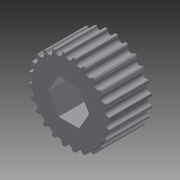
# Autodesk Inventor part: 24t Tooth Pulley .375 Hex Bore 3mm GT2
Saved by Autodesk Inventor 2013 (Build 170138000, 138)
## iProperties
Created: 2013-04-02
Part Number: 24t Tooth Pulley .375 Hex Bore 3mm GT2
Material: Generic
Document SubType Name: Modeling
Designer: mvarma
Density: 1 g/cm^3
Author: mvarma
Autodesk Inventor part; units mm, degrees
ref_plane "YZ Plane" through (0, 0, 0) normal (1, 0, 0) x (0, 1, 0)
ref_plane "XZ Plane" through (0, 0, 0) normal (0, 1, 0) x (-1, 0, 0)
sketch "Sketch1" plane through (0, 0, 0) normal (0, 0, 1) x (1, 0, 0)
  arc A0 (4.5197, -1.1407) -> (6.1695, -2.0932) centre (5.437, -1.4568) ccw
  arc A1 (4.5197, -1.1407) -> (4.3966, -0.6901) centre (4.2781, -0.9646) ccw
  arc A2 (4.3966, -0.6901) -> (4.0923, -0.564) centre (0, -10.8741) ccw
  arc A3 (4.0923, -0.564) -> (3.6866, -0.7956) centre (3.982, -0.8419) ccw
  arc A4 (1.8465, -0.3026) -> (3.6866, -0.7956) centre (2.8144, -0.3705) ccw
  arc A5 (1.8465, -0.3026) -> (1.611, 0.1008) centre (1.5675, -0.195) ccw
  arc A6 (1.611, 0.1008) -> (1.2844, 0.1438) centre (0, -10.8741) ccw
  arc A7 (1.2844, 0.1438) -> (0.9525, -0.1849) centre (1.2498, -0.1532) ccw
  arc A8 (-0.9525, -0.1849) -> (0.9525, -0.1849) centre (0, 0) ccw
  arc A9 (-0.9525, -0.1849) -> (-1.2844, 0.1438) centre (-1.2498, -0.1532) ccw
  arc A10 (-1.2844, 0.1438) -> (-1.611, 0.1008) centre (0, -10.8741) ccw
  arc A11 (-1.611, 0.1008) -> (-1.8465, -0.3026) centre (-1.5675, -0.195) ccw
  arc A12 (-3.6866, -0.7956) -> (-1.8465, -0.3026) centre (-2.8144, -0.3705) ccw
  arc A13 (-3.6866, -0.7956) -> (-4.0923, -0.564) centre (-3.982, -0.8419) ccw
  arc A14 (-4.0923, -0.564) -> (-4.3966, -0.6901) centre (0, -10.8741) ccw
  arc A15 (-4.3966, -0.6901) -> (-4.5197, -1.1407) centre (-4.2781, -0.9646) ccw
  arc A16 (-6.1695, -2.0932) -> (-4.5197, -1.1407) centre (-5.437, -1.4568) ccw
  arc A17 (-6.1695, -2.0932) -> (-6.6213, -1.9745) centre (-6.4428, -2.2144) ccw
  arc A18 (-6.6213, -1.9745) -> (-6.8826, -2.175) centre (0, -10.8741) ccw
  arc A19 (-6.8826, -2.175) -> (-6.8849, -2.6422) centre (-6.6971, -2.4095) ccw
  arc A20 (-8.2319, -3.9892) -> (-6.8849, -2.6422) centre (-7.6891, -3.1849) ccw
  arc A21 (-8.2319, -3.9892) -> (-8.6991, -3.9915) centre (-8.4646, -4.177) ccw
  arc A22 (-8.6991, -3.9915) -> (-8.8996, -4.2528) centre (0, -10.8741) ccw
  arc A23 (-8.8996, -4.2528) -> (-8.7808, -4.7046) centre (-8.6597, -4.4312) ccw
  arc A24 (-9.7333, -6.3544) -> (-8.7808, -4.7046) centre (-9.4172, -5.437) ccw
  arc A25 (-9.7333, -6.3544) -> (-10.184, -6.4775) centre (-9.9095, -6.596) ccw
  arc A26 (-10.184, -6.4775) -> (-10.31, -6.7818) centre (0, -10.8741) ccw
  arc A27 (-10.31, -6.7818) -> (-10.0784, -7.1875) centre (-10.0321, -6.8921) ccw
  arc A28 (-10.5715, -9.0275) -> (-10.0784, -7.1875) centre (-10.5035, -8.0596) ccw
  arc A29 (-10.5715, -9.0275) -> (-10.9749, -9.2631) centre (-10.6791, -9.3065) ccw
  arc A30 (-10.9749, -9.2631) -> (-11.0179, -9.5896) centre (0, -10.8741) ccw
  arc A31 (-11.0179, -9.5896) -> (-10.6892, -9.9216) centre (-10.7209, -9.6242) ccw
  arc A32 (-10.6892, -11.8266) -> (-10.6892, -9.9216) centre (-10.8741, -10.8741) ccw
  arc A33 (-10.6892, -11.8266) -> (-11.0179, -12.1585) centre (-10.7209, -12.1239) ccw
  arc A34 (-11.0179, -12.1585) -> (-10.9749, -12.485) centre (0, -10.8741) ccw
  arc A35 (-10.9749, -12.485) -> (-10.5715, -12.7206) centre (-10.6791, -12.4416) ccw
  arc A36 (-10.0784, -14.5607) -> (-10.5715, -12.7206) centre (-10.5035, -13.6885) ccw
  arc A37 (-10.0784, -14.5607) -> (-10.31, -14.9664) centre (-10.0321, -14.8561) ccw
  arc A38 (-10.31, -14.9664) -> (-10.184, -15.2707) centre (0, -10.8741) ccw
  arc A39 (-10.184, -15.2707) -> (-9.7333, -15.3938) centre (-9.9095, -15.1521) ccw
  arc A40 (-8.7808, -17.0435) -> (-9.7333, -15.3938) centre (-9.4172, -16.3111) ccw
  arc A41 (-8.7808, -17.0435) -> (-8.8996, -17.4954) centre (-8.6597, -17.3169) ccw
  arc A42 (-8.8996, -17.4954) -> (-8.6991, -17.7566) centre (0, -10.8741) ccw
  arc A43 (-8.6991, -17.7566) -> (-8.2319, -17.7589) centre (-8.4646, -17.5711) ccw
  arc A44 (-6.8849, -19.106) -> (-8.2319, -17.7589) centre (-7.6891, -18.5632) ccw
  arc A45 (-6.8849, -19.106) -> (-6.8826, -19.5731) centre (-6.6971, -19.3386) ccw
  arc A46 (-6.8826, -19.5731) -> (-6.6213, -19.7736) centre (0, -10.8741) ccw
  arc A47 (-6.6213, -19.7736) -> (-6.1695, -19.6549) centre (-6.4428, -19.5337) ccw
  arc A48 (-4.5197, -20.6074) -> (-6.1695, -19.6549) centre (-5.437, -20.2913) ccw
  arc A49 (-4.5197, -20.6074) -> (-4.3966, -21.058) centre (-4.2781, -20.7835) ccw
  arc A50 (-4.3966, -21.058) -> (-4.0923, -21.1841) centre (0, -10.8741) ccw
  arc A51 (-4.0923, -21.1841) -> (-3.6866, -20.9525) centre (-3.982, -20.9062) ccw
  arc A52 (-1.8465, -21.4455) -> (-3.6866, -20.9525) centre (-2.8144, -21.3776) ccw
  arc A53 (-1.8465, -21.4455) -> (-1.611, -21.849) centre (-1.5675, -21.5531) ccw
  arc A54 (-1.611, -21.849) -> (-1.2844, -21.8919) centre (0, -10.8741) ccw
  arc A55 (-1.2844, -21.8919) -> (-0.9525, -21.5632) centre (-1.2498, -21.595) ccw
  arc A56 (0.9525, -21.5632) -> (-0.9525, -21.5632) centre (0, -21.7481) ccw
  arc A57 (0.9525, -21.5632) -> (1.2844, -21.8919) centre (1.2498, -21.595) ccw
  arc A58 (1.2844, -21.8919) -> (1.611, -21.849) centre (0, -10.8741) ccw
  arc A59 (1.611, -21.849) -> (1.8465, -21.4455) centre (1.5675, -21.5531) ccw
  arc A60 (3.6866, -20.9525) -> (1.8465, -21.4455) centre (2.8144, -21.3776) ccw
  arc A61 (3.6866, -20.9525) -> (4.0923, -21.1841) centre (3.982, -20.9062) ccw
  arc A62 (4.0923, -21.1841) -> (4.3966, -21.058) centre (0, -10.8741) ccw
  arc A63 (4.3966, -21.058) -> (4.5197, -20.6074) centre (4.2781, -20.7835) ccw
  arc A64 (6.1695, -19.6549) -> (4.5197, -20.6074) centre (5.437, -20.2913) ccw
  arc A65 (6.1695, -19.6549) -> (6.6213, -19.7736) centre (6.4428, -19.5337) ccw
  arc A66 (6.6213, -19.7736) -> (6.8826, -19.5731) centre (0, -10.8741) ccw
  arc A67 (6.8826, -19.5731) -> (6.8849, -19.106) centre (6.6971, -19.3386) ccw
  arc A68 (8.2319, -17.7589) -> (6.8849, -19.106) centre (7.6891, -18.5632) ccw
  arc A69 (8.2319, -17.7589) -> (8.6991, -17.7566) centre (8.4646, -17.5711) ccw
  arc A70 (8.6991, -17.7566) -> (8.8996, -17.4954) centre (0, -10.8741) ccw
  arc A71 (8.8996, -17.4954) -> (8.7808, -17.0435) centre (8.6597, -17.3169) ccw
  arc A72 (9.7333, -15.3938) -> (8.7808, -17.0435) centre (9.4172, -16.3111) ccw
  arc A73 (9.7333, -15.3938) -> (10.184, -15.2707) centre (9.9095, -15.1521) ccw
  arc A74 (10.184, -15.2707) -> (10.31, -14.9664) centre (0, -10.8741) ccw
  arc A75 (10.31, -14.9664) -> (10.0784, -14.5607) centre (10.0321, -14.8561) ccw
  arc A76 (10.5715, -12.7206) -> (10.0784, -14.5607) centre (10.5035, -13.6885) ccw
  arc A77 (10.5715, -12.7206) -> (10.9749, -12.485) centre (10.6791, -12.4416) ccw
  arc A78 (10.9749, -12.485) -> (11.0179, -12.1585) centre (0, -10.8741) ccw
  arc A79 (11.0179, -12.1585) -> (10.6892, -11.8266) centre (10.7209, -12.1239) ccw
  arc A80 (10.6892, -9.9216) -> (10.6892, -11.8266) centre (10.8741, -10.8741) ccw
  arc A81 (10.6892, -9.9216) -> (11.0179, -9.5896) centre (10.7209, -9.6242) ccw
  arc A82 (11.0179, -9.5896) -> (10.9749, -9.2631) centre (0, -10.8741) ccw
  arc A83 (10.9749, -9.2631) -> (10.5715, -9.0275) centre (10.6791, -9.3065) ccw
  arc A84 (10.0784, -7.1875) -> (10.5715, -9.0275) centre (10.5035, -8.0596) ccw
  arc A85 (10.0784, -7.1875) -> (10.31, -6.7818) centre (10.0321, -6.8921) ccw
  arc A86 (10.31, -6.7818) -> (10.184, -6.4775) centre (0, -10.8741) ccw
  arc A87 (10.184, -6.4775) -> (9.7333, -6.3544) centre (9.9095, -6.596) ccw
  arc A88 (8.7808, -4.7046) -> (9.7333, -6.3544) centre (9.4172, -5.437) ccw
  arc A89 (8.7808, -4.7046) -> (8.8996, -4.2528) centre (8.6597, -4.4312) ccw
  arc A90 (8.8996, -4.2528) -> (8.6991, -3.9915) centre (0, -10.8741) ccw
  arc A91 (8.6991, -3.9915) -> (8.2319, -3.9892) centre (8.4646, -4.177) ccw
  arc A92 (6.8849, -2.6422) -> (8.2319, -3.9892) centre (7.6891, -3.1849) ccw
  arc A93 (6.8849, -2.6422) -> (6.8826, -2.175) centre (6.6971, -2.4095) ccw
  arc A94 (6.8826, -2.175) -> (6.6213, -1.9745) centre (0, -10.8741) ccw
  arc A95 (6.6213, -1.9745) -> (6.1695, -2.0932) centre (6.4428, -2.2144) ccw
  line L0 (-5.4993, -10.8741) -> (-2.7496, -6.1116)
  line L1 (-2.7496, -6.1116) -> (2.7496, -6.1116)
  line L2 (2.7496, -6.1116) -> (5.4993, -10.8741)
  line L3 (5.4993, -10.8741) -> (2.7496, -15.6366)
  line L4 (2.7496, -15.6366) -> (-2.7496, -15.6366)
  line L5 (-2.7496, -15.6366) -> (-5.4993, -10.8741)
  dimension "d0" = 9.525
  constraints: 192 point on circle, 96 centre point, 12 end point, 1 coincident, 1 horizontal, 302 other
  measures "d0" distance between parallel lines of L4 L1
extrude "Extrusion1" add sketch "Sketch1" along normal blind 11.43
ref_plane "Work Plane1" through (0, 0, 5.715) normal (0, 0, -1) x (-1, 0, 0)
body "Solid1"
